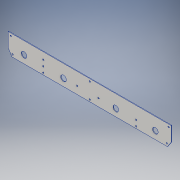
# Autodesk Inventor part: OutsidePlate2
Saved by Autodesk Inventor 2016 (Build 200138000, 138)
## iProperties
Created: 2017-01-21
Part Number: OutsidePlate2
Material: Aluminum 6061
Document SubType Name: Modeling
Designer: hamblettk
Density: 2.7 g/cm^3
Appearance: Aluminum - Flat
Mass: 687.372 g
Surface Area: 1683.05 cm^2
Volume: 254.582 cm^3
Author: hamblettk
Autodesk Inventor part; units mm, degrees
ref_plane "YZ Plane" through (0, 0, 0) normal (1, 0, 0) x (0, 1, 0)
ref_plane "XZ Plane" through (0, 0, 0) normal (0, 1, 0) x (-1, 0, 0)
ref_plane "XY Plane" through (0, 0, 0) normal (0, 0, 1) x (1, 0, 0)
sketch "Sketch1" plane through (0, 0, 0) normal (0, 0, 1) x (1, 0, 0)
  line L0 (0, 0) -> (850.9, 0)
  line L1 (850.9, 0) -> (850.9, 76.2)
  line L2 (850.9, 76.2) -> (0, 76.2)
  line L3 (0, 76.2) -> (0, 0)
  dimension "d0" = 850.9
  dimension "d1" = 76.2
  constraints: 8 end point, 2 parallel, 1 horizontal, 1 perpendicular
  measures "d0" distance of L2.end L1.end
  measures "d1" distance of L1.end L0.end
extrude "Extrusion1" add sketch "Sketch1" along normal blind 3.175
sketch "Sketch4" plane through (0, 0, 3.175) normal (0, 0, 1) x (1, 0, 0)
  line L0 (0, 0) -> (0, 38.1)
  line L1 (0, 76.2) -> (0, 0) projected
  line L2 (0, 0) -> (25.4, 0)
  line L3 (0, 0) -> (850.9, 0) projected
  line L4 (25.4, 0) -> (0, 38.1)
  line L5 (850.9, 0) -> (825.5, 0)
  line L6 (850.9, 0) -> (850.9, 38.1)
  line L7 (850.9, 0) -> (850.9, 76.2) projected
  line L8 (850.9, 38.1) -> (825.5, 0)
  line L9 (0, 38.1) -> (0, 36.5125)
  circle A0 centre (292.9509, 36.5125) radius 14.2875
  circle A1 centre (557.9491, 36.5125) radius 14.2875
  circle A2 centre (757.9743, 39.6875) radius 14.2875
  circle A3 centre (92.9257, 39.6875) radius 14.2875
  dimension "d24" = 38.1
  dimension "d26" = 25.4
  dimension "d27" = 38.1
  dimension "d33" = 28.575
  dimension "d34" = 28.575
  dimension "d38" = 28.575
  dimension "d39" = 28.575
  constraints: 14 end point, 4 centre point, 3 point on line, 2 midpoint
  measures "d24" distance of L0.start L0.end
  measures "d26" distance of L3.end L5.end
  measures "d27" distance of L3.end L6.end
  measures "d33" diameter of A0
  measures "d34" diameter of A1
  measures "d38" diameter of A2
  measures "d39" diameter of A3
extrude "Extrusion3" cut sketch "Sketch4" against normal blind 3.175
sketch "Sketch5" plane through (0, 0, 3.175) normal (0, 0, 1) x (1, 0, 0)
  line L0 (850.9, 76.2) -> (0, 76.2) projected
  line L1 (0, 76.2) -> (425.45, 76.2)
  circle A0 centre (425.45, 66.675) radius 3.5687
  circle A1 centre (425.45, 9.525) radius 3.5687
  line L2 (25.4, 0) -> (825.5, 0) projected
  line L3 (0, 76.2) -> (190.5, 76.2)
  circle A2 centre (190.5, 66.675) radius 3.5687
  circle A3 centre (190.5, 9.525) radius 3.5687
  circle A4 centre (190.5, 38.1) radius 3.5687
  line L4 (850.9, 38.1) -> (850.9, 76.2) projected
  line L5 (850.9, 76.2) -> (660.4, 76.2)
  circle A5 centre (660.4, 66.675) radius 3.5687
  circle A6 centre (660.4, 9.525) radius 3.5687
  circle A7 centre (660.4, 38.1) radius 3.5687
  circle A8 centre (838.2, 63.5) radius 3.5687
  circle A9 centre (12.7, 63.5) radius 3.5687
  line L6 (0, 76.2) -> (0, 38.1) projected
  circle A10 centre (34.925, 12.7) radius 3.5687
  circle A11 centre (815.975, 12.7) radius 3.5687
  point P0 (0, 0)
  dimension "d42" = 425.45
  dimension "d43" = 7.1374
  dimension "d44" = 9.525
  dimension "d45" = 7.1374
  dimension "d46" = 9.525
  dimension "d47" = 190.5
  dimension "d48" = 7.1374
  dimension "d49" = 9.525
  dimension "d50" = 7.1374
  dimension "d51" = 9.525
  dimension "d52" = 7.1374
  dimension "d53" = 38.1
  dimension "d54" = 190.5
  dimension "d55" = 7.1374
  dimension "d56" = 9.525
  dimension "d57" = 7.1374
  dimension "d58" = 9.525
  dimension "d59" = 7.1374
  dimension "d60" = 38.1
  dimension "d61" = 7.1374
  dimension "d62" = 12.7
  dimension "d63" = 12.7
  dimension "d64" = 7.1374
  dimension "d65" = 12.7
  dimension "d66" = 12.7
  dimension "d67" = 7.1374
  dimension "d69" = 12.7
  dimension "d70" = 9.525
  dimension "d71" = 7.1374
  dimension "d72" = 12.7
  dimension "d73" = 9.525
  constraints: 12 centre point, 6 end point, 2 point on line, 1 midpoint
  measures "d42" distance of L0.end L1.end
  measures "d43" diameter of A0
  measures "d44" distance from line of L0 A0.centre
  measures "d45" diameter of A1
  measures "d46" distance from line of L2 A1.centre
  measures "d47" distance of L0.end L3.end
  measures "d48" diameter of A2
  measures "d49" distance from line of L0 A2.centre
  measures "d50" diameter of A3
  measures "d51" distance from line of L2 A3.centre
  measures "d52" diameter of A4
  measures "d53" distance from line of L2 A4.centre
  measures "d54" distance of L0.start L5.end
  measures "d55" diameter of A5
  measures "d56" distance from line of L0 A5.centre
  measures "d57" diameter of A6
  measures "d58" distance from line of L2 A6.centre
  measures "d59" diameter of A7
  measures "d60" distance from line of L2 A7.centre
  measures "d61" diameter of A8
  measures "d62" distance from line of L0 A8.centre
  measures "d63" distance from line of L4 A8.centre
  measures "d64" diameter of A9
  measures "d65" distance from line of L1 A9.centre
  measures "d66" distance from line of L6 A9.centre
  measures "d67" diameter of A10
  measures "d69" distance from line of L2 A10.centre
  measures "d70" horizontal distance of L2.start A10.centre
  measures "d71" diameter of A11
  measures "d72" distance from line of L2 A11.centre
  measures "d73" horizontal distance of L2.end A11.centre
extrude "Extrusion4" cut sketch "Sketch5" against normal blind 3.175
sketch "Sketch6" plane through (0, 0, 3.175) normal (0, 0, 1) x (1, 0, 0)
  circle A0 centre (361.95, 38.1) radius 3.5687
  circle A1 centre (469.9, 38.1) radius 3.5687
  line L0 (850.9, 76.2) -> (0, 76.2) projected
  circle A2 centre (292.9509, 36.5125) radius 14.2875 projected
  line L1 (0, 76.2) -> (0, 38.1) projected
  line L2 (850.9, 38.1) -> (850.9, 76.2) projected
  point P0 (0, 0)
  dimension "d76" = 7.1374
  dimension "d77" = 7.1374
  dimension "d78" = 38.1
  dimension "d79" = 38.1
  dimension "d82" = 381
  dimension "d83" = 361.95
  constraints: 2 centre point
  measures "d76" diameter of A0
  measures "d77" diameter of A1
  measures "d78" distance from line of L0 A1.centre
  measures "d79" distance from line of L0 A0.centre
  measures "d82" distance from line of L2 A1.centre
  measures "d83" distance from line of L1 A0.centre
extrude "Extrusion6" cut sketch "Sketch6" against normal blind 25.4 contours A0 | A1
sketch "Sketch7" plane through (0, 76.2, 0) normal (0, 1, 0) x (1, 0, 0)
  line L0 (850.9, 0) -> (0, 0) projected
  line L1 (0, 0) -> (0, -3.175) projected
  line L2 (850.9, -3.175) -> (0, -3.175) projected
  line L3 (850.9, 0) -> (850.9, -3.175) projected
extrude "Extrusion7" add sketch "Sketch7" along normal blind 25.4
sketch "Sketch8" plane through (0, 0, 3.175) normal (0, 0, 1) x (1, 0, 0)
  circle A0 centre (12.7, 63.5) radius 3.5687 projected
  circle A1 centre (838.2, 63.5) radius 3.5687 projected
  circle A2 centre (425.45, 66.675) radius 3.5687 projected
  point P0 (0, 0)
extrude "Extrusion9" add sketch "Sketch8" against normal blind 3.175
sketch "Sketch9" plane through (0, 0, 3.175) normal (0, 0, 1) x (1, 0, 0)
  circle A0 centre (12.7, 88.9) radius 3.5687
  line L0 (0, 101.6) -> (850.9, 101.6) projected
  line L1 (0, 38.1) -> (0, 101.6) projected
  circle A1 centre (838.2, 88.9) radius 3.5687
  line L2 (850.9, 38.1) -> (850.9, 101.6) projected
  circle A2 centre (425.45, 88.9) radius 3.5687
  point P0 (0, 0)
  dimension "d95" = 7.1374
  dimension "d96" = 12.7
  dimension "d97" = 12.7
  dimension "d98" = 7.1374
  dimension "d99" = 12.7
  dimension "d100" = 12.7
  dimension "d101" = 7.1374
  constraints: 3 centre point
  measures "d95" diameter of A0
  measures "d96" distance from line of L0 A0.centre
  measures "d97" distance from line of L1 A0.centre
  measures "d98" diameter of A1
  measures "d99" distance from line of L0 A1.centre
  measures "d100" distance from line of L2 A1.centre
  measures "d101" diameter of A2
extrude "Extrusion10" cut sketch "Sketch9" against normal blind 3.175
sketch "Sketch10" plane through (0, 0, 3.175) normal (0, 0, 1) x (1, 0, 0)
  line L0 (0, 38.1) -> (0, 101.6) projected
  line L1 (0, 101.6) -> (12.7, 101.6)
  line L2 (0, 101.6) -> (850.9, 101.6) projected
  line L3 (12.7, 101.6) -> (12.7, 19.05)
  line L4 (0, 38.1) -> (25.4, 0) projected
  line L5 (850.9, 101.6) -> (838.2, 101.6)
  line L6 (838.2, 101.6) -> (838.2, 19.05)
  line L7 (825.5, 0) -> (850.9, 38.1) projected
  line L8 (838.2, 19.05) -> (850.9, 38.1)
  line L9 (850.9, 38.1) -> (850.9, 101.6) projected
  line L10 (850.9, 101.6) -> (850.9, 38.1)
  line L11 (12.7, 19.05) -> (0, 38.1)
  line L12 (0, 101.6) -> (0, 38.1)
  point P0 (0, 0)
  dimension "d104" = 12.7
  dimension "d105" = 12.7
  constraints: 16 end point, 2 collinear, 2 midpoint, 2 point on line, 2 vertical
  measures "d104" distance of L0.end L1.end
  measures "d105" distance of L2.end L5.end
extrude "Extrusion11" cut sketch "Sketch10" against normal blind 25.4
sketch "Sketch11" plane through (0, 0, 3.175) normal (0, 0, 1) x (1, 0, 0)
  arc A0 (12.7, 85.3313) -> (12.7, 92.4687) centre (12.7, 88.9) ccw projected
  line L0 (12.7, 92.4687) -> (12.7, 85.3313)
  arc A1 (838.2, 92.4687) -> (838.2, 85.3313) centre (838.2, 88.9) ccw projected
  line L1 (838.2, 92.4687) -> (838.2, 85.3313)
  point P0 (0, 0)
  constraints: 4 end point, 2 vertical
extrude "Extrusion12" add sketch "Sketch11" against normal blind 3.175
sketch "Sketch12" plane through (0, 0, 3.175) normal (0, 0, 1) x (1, 0, 0)
  line L0 (25.4, 0) -> (825.5, 0) projected
  line L1 (25.4, 0) -> (31.75, 0)
  line L2 (31.75, 0) -> (12.7, 30.4376)
  line L3 (12.7, 19.05) -> (12.7, 101.6) projected
  line L4 (12.7, 30.4376) -> (12.7, 19.05)
  line L5 (25.4, 0) -> (12.7, 19.05) projected
  line L6 (12.7, 19.05) -> (25.4, 0)
  line L7 (25.4, 0) -> (31.75, 0)
  line L8 (25.4, 0) -> (12.7, 19.05)
  line L9 (838.2, 19.05) -> (825.5, 0) projected
  line L10 (825.5, 0) -> (819.15, 0)
  line L11 (819.15, 0) -> (838.2, 28.575)
  line L12 (838.2, 101.6) -> (838.2, 19.05) projected
  line L13 (838.2, 28.575) -> (838.2, 19.05)
  line L14 (838.2, 19.05) -> (825.5, 0)
  point P0 (0, 0)
  dimension "d111" = 6.35
  dimension "d113" = 6.35
  constraints: 20 end point, 4 collinear, 4 point on line, 1 parallel, 1 perpendicular
  measures "d111" distance of L0.start L1.end
  measures "d113" distance of L0.end L10.end
extrude "Extrusion13" cut sketch "Sketch12" against normal blind 3.175
sketch "Sketch13" plane through (0, 0, 3.175) normal (0, 0, 1) x (1, 0, 0)
  circle A0 centre (25.4, 88.9) radius 3.5687
  line L0 (12.7, 101.6) -> (838.2, 101.6) projected
  line L1 (12.7, 101.6) -> (12.7, 30.4376) projected
  circle A1 centre (825.5, 88.9) radius 3.5687
  line L2 (838.2, 101.6) -> (838.2, 28.575) projected
  point P0 (0, 0)
  dimension "d116" = 7.1374
  dimension "d117" = 12.7
  dimension "d118" = 12.7
  dimension "d119" = 7.1374
  dimension "d120" = 12.7
  dimension "d121" = 12.7
  constraints: 2 centre point
  measures "d116" diameter of A0
  measures "d117" distance from line of L0 A0.centre
  measures "d118" distance from line of L1 A0.centre
  measures "d119" diameter of A1
  measures "d120" distance from line of L0 A1.centre
  measures "d121" distance from line of L2 A1.centre
extrude "Extrusion14" cut sketch "Sketch13" against normal blind 3.175
sketch "Sketch14" plane through (0, 0, 3.175) normal (0, 0, 1) x (1, 0, 0)
  circle A0 centre (660.4, 66.675) radius 3.5687 projected
  circle A1 centre (660.4, 38.1) radius 3.5687 projected
  point P0 (0, 0)
  dimension "d124" = 28.575
  measures "d124" distance of A1.centre A0.centre
extrude "Extrusion15" add sketch "Sketch14" against normal blind 3.175 contours A0
body "Solid1"
